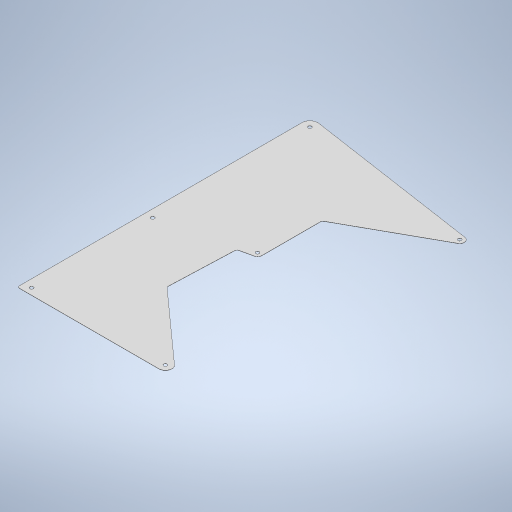
# Autodesk Inventor part: base_main_pcb_full_itr2
Saved by Autodesk Inventor 2024 (Build 280153000, 153)
## iProperties
Created: 2026-03-21
Part Number: base_main_pcb_full_itr2
Material: Generic
Document SubType Name: Modeling
Designer: schar
Density: 1 g/cm^3
Appearance: Default
Author: schar
Autodesk Inventor part; units mm, degrees
ref_plane "YZ Plane" through (0, 0, 0) normal (1, 0, 0) x (0, 1, 0)
ref_plane "XZ Plane" through (0, 0, 0) normal (0, 1, 0) x (-1, 0, 0)
ref_plane "Work Plane1" through (-205, 0.2, 0) normal (0, 1, 0) x (1, 0, 0)
sketch "Sketch1" plane through (-205, 0.2, 0) normal (0, 1, 0) x (1, 0, 0)
  circle A0 centre (135.6, -283.785) radius 1.675 projected
  circle A1 centre (135.6, -283.785) radius 6.215
  line L0 (0, -290) -> (155, -290) projected
  circle A2 centre (7.5, -283.785) radius 1.675 projected
  circle A3 centre (7.5, -283.785) radius 6.215
  circle A4 centre (7.5, -167.775) radius 1.675 projected
  circle A5 centre (7.5, -167.775) radius 7.5
  line L1 (0, 0) -> (0, -290) projected
  circle A6 centre (86.5, -146.525) radius 1.675 projected
  circle A7 centre (86.5, -146.525) radius 4.5
  circle A8 centre (7.5, -17.325) radius 1.675 projected
  circle A9 centre (7.5, -17.325) radius 7.5068
  circle A10 centre (172.5, -38.875) radius 1.675 projected
  circle A11 centre (172.5, -38.875) radius 4.5
  line L2 (14.9987, -167.6345) -> (86.5, -151.025)
  line L3 (172.5, -34.375) -> (8.6087, -9.9005)
  line L4 (91, -146.525) -> (91, -89.2982)
  line L5 (91, -89.2982) -> (174.6853, -42.8088)
  line L6 (140.4129, -279.8528) -> (14.9987, -167.6345)
  line L7 (135.6, -290) -> (7.5, -290)
  line L8 (7.5, -290) -> (0, -290)
  line L9 (0, -290) -> (0, -167.775)
  line L10 (0, -167.775) -> (0, -17.6452)
  line L11 (8.6087, -9.9005) -> (8.6087, 0)
  line L12 (8.6087, 0) -> (0, 0)
  line L13 (0, 0) -> (0, -17.6452)
  line L14 (73.9664, -153.9365) -> (71.55, -218.2356)
  point P0 (205, 0)
  point P1 (0, -17.0048)
  dimension "d1" = 9
  dimension "d2" = 9
  constraints: 26 end point, 10 point on circle, 6 coincident, 6 point on line, 5 centre point, 4 tangent, 2 horizontal, 2 perpendicular, 1 collinear, 1 parallel, 1 vertical, 1 vertical alignment, 2 other
  measures "d1" diameter of A7
  measures "d2" diameter of A11
extrude "Extrusion1" add sketch "Sketch1" along normal blind 0.2 contours A1 L6 | A3 | L0 L1 A5 L6 A1 | L6 L2 L14 | A5 | A5 L1 A9 L3 A11 L5 L4 A7 L2 | A7 | L1 A9 | A11 picked at (138.7473, -280.3645) picked at (7.7088, -11.8041)
fillet "Fillet1" radius 2 4 edges at (-133.45, 0.3, 218.2356) (-114, 0.3, 89.2982) (-205, 0.3, 290) (-131.0336, 0.3, 153.9365)
body "Solid2"
